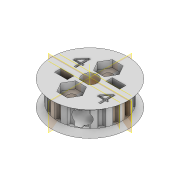
# Autodesk Inventor part: 18 tooth .2 pitch .25 wide belt pulley .25 D bore base
Saved by Autodesk Inventor 2020 (Build 240168000, 168)
## iProperties
Created: 2020-01-17
Part Number: 18 tooth .2 pitch .25 wide belt pulley .25 D bore base
Material: Generic
Document SubType Name: Modeling
Designer: ball
Density: 1 g/cm^3
Appearance: Default
Author: ball
Autodesk Inventor part; units mm, degrees
note: some values were not read from the file. Chosen so that the rebuilt part matches the saved one: direction of "Emboss1".
ref_plane "XZ Plane" through (0, 0, 0) normal (0, 1, 0) x (-1, 0, 0)
sketch "Sketch1" plane through (0, 0, 0) normal (0, 1, 0) x (-1, 0, 0)
  arc A0 (-6.0094, 12.7604) -> (-8.0461, 11.5845) centre (0, 0) ccw
  line L0 (-7.6834, 10.231) -> (-8.0461, 11.5845)
  line L1 (-8.7413, 9.3433) -> (-7.6834, 10.231)
  line L2 (-10.0113, 9.9355) -> (-8.7413, 9.3433)
  arc A1 (-10.0113, 9.9355) -> (-11.523, 8.134) centre (0, 0) ccw
  line L3 (-10.7193, 6.9861) -> (-11.523, 8.134)
  line L4 (-11.4098, 5.7901) -> (-10.7193, 6.9861)
  line L5 (-12.8057, 5.9122) -> (-11.4098, 5.7901)
  arc A2 (-12.8057, 5.9122) -> (-13.6101, 3.7023) centre (0, 0) ccw
  line L6 (-12.4622, 2.8986) -> (-13.6101, 3.7023)
  line L7 (-12.702, 1.5386) -> (-12.4622, 2.8986)
  line L8 (-14.0555, 1.1759) -> (-12.702, 1.5386)
  arc A3 (-14.0555, 1.1759) -> (-14.0555, -1.1759) centre (0, 0) ccw
  line L9 (-12.702, -1.5386) -> (-14.0555, -1.1759)
  line L10 (-12.4622, -2.8986) -> (-12.702, -1.5386)
  line L11 (-13.6101, -3.7023) -> (-12.4622, -2.8986)
  arc A4 (-13.6101, -3.7023) -> (-12.8057, -5.9122) centre (0, 0) ccw
  line L12 (-11.4098, -5.7901) -> (-12.8057, -5.9122)
  line L13 (-10.7193, -6.9861) -> (-11.4098, -5.7901)
  line L14 (-11.523, -8.134) -> (-10.7193, -6.9861)
  arc A5 (-11.523, -8.134) -> (-10.0113, -9.9355) centre (0, 0) ccw
  line L15 (-8.7413, -9.3433) -> (-10.0113, -9.9355)
  line L16 (-7.6834, -10.231) -> (-8.7413, -9.3433)
  line L17 (-8.0461, -11.5845) -> (-7.6834, -10.231)
  arc A6 (-8.0461, -11.5845) -> (-6.0094, -12.7604) centre (0, 0) ccw
  line L18 (-5.0186, -11.7695) -> (-6.0094, -12.7604)
  line L19 (-3.7209, -12.2419) -> (-5.0186, -11.7695)
  line L20 (-3.5987, -13.6378) -> (-3.7209, -12.2419)
  arc A7 (-3.5987, -13.6378) -> (-1.2827, -14.0462) centre (0, 0) ccw
  line L21 (-0.6905, -12.7762) -> (-1.2827, -14.0462)
  line L22 (0.6905, -12.7762) -> (-0.6905, -12.7762)
  line L23 (1.2827, -14.0462) -> (0.6905, -12.7762)
  arc A8 (1.2827, -14.0462) -> (3.5987, -13.6378) centre (0, 0) ccw
  line L24 (3.7209, -12.2419) -> (3.5987, -13.6378)
  line L25 (5.0186, -11.7695) -> (3.7209, -12.2419)
  line L26 (6.0094, -12.7604) -> (5.0186, -11.7695)
  arc A9 (6.0094, -12.7604) -> (8.0461, -11.5845) centre (0, 0) ccw
  line L27 (7.6834, -10.231) -> (8.0461, -11.5845)
  line L28 (8.7413, -9.3433) -> (7.6834, -10.231)
  line L29 (10.0113, -9.9355) -> (8.7413, -9.3433)
  arc A10 (10.0113, -9.9355) -> (11.523, -8.134) centre (0, 0) ccw
  line L30 (10.7193, -6.9861) -> (11.523, -8.134)
  line L31 (11.4098, -5.7901) -> (10.7193, -6.9861)
  line L32 (12.8057, -5.9122) -> (11.4098, -5.7901)
  arc A11 (12.8057, -5.9122) -> (13.6101, -3.7023) centre (0, 0) ccw
  line L33 (12.4622, -2.8986) -> (13.6101, -3.7023)
  line L34 (12.702, -1.5386) -> (12.4622, -2.8986)
  line L35 (14.0555, -1.1759) -> (12.702, -1.5386)
  arc A12 (14.0555, -1.1759) -> (14.0555, 1.1759) centre (0, 0) ccw
  line L36 (12.702, 1.5386) -> (14.0555, 1.1759)
  line L37 (12.4622, 2.8986) -> (12.702, 1.5386)
  line L38 (13.6101, 3.7023) -> (12.4622, 2.8986)
  arc A13 (13.6101, 3.7023) -> (12.8057, 5.9122) centre (0, 0) ccw
  line L39 (11.4098, 5.7901) -> (12.8057, 5.9122)
  line L40 (10.7193, 6.9861) -> (11.4098, 5.7901)
  line L41 (11.523, 8.134) -> (10.7193, 6.9861)
  arc A14 (11.523, 8.134) -> (10.0113, 9.9355) centre (0, 0) ccw
  line L42 (8.7413, 9.3433) -> (10.0113, 9.9355)
  line L43 (7.6834, 10.231) -> (8.7413, 9.3433)
  line L44 (8.0461, 11.5845) -> (7.6834, 10.231)
  arc A15 (8.0461, 11.5845) -> (6.0094, 12.7604) centre (0, 0) ccw
  line L45 (5.0186, 11.7695) -> (6.0094, 12.7604)
  line L46 (3.7209, 12.2419) -> (5.0186, 11.7695)
  line L47 (3.5987, 13.6378) -> (3.7209, 12.2419)
  arc A16 (3.5987, 13.6378) -> (1.2827, 14.0462) centre (0, 0) ccw
  line L48 (0.6905, 12.7762) -> (1.2827, 14.0462)
  line L49 (-0.6905, 12.7762) -> (0.6905, 12.7762)
  line L50 (-1.2827, 14.0462) -> (-0.6905, 12.7762)
  arc A17 (-1.2827, 14.0462) -> (-3.5987, 13.6378) centre (0, 0) ccw
  line L51 (-3.7209, 12.2419) -> (-3.5987, 13.6378)
  line L52 (-5.0186, 11.7695) -> (-3.7209, 12.2419)
  line L53 (-6.0094, 12.7604) -> (-5.0186, 11.7695)
  constraints: 108 end point, 36 point on circle, 18 centre point
extrude "Extrusion1" add sketch "Sketch1" along normal blind 3.4925 and the other way blind 3.4925
sketch "Sketch6" plane through (0, 0, 0) normal (0, 0, 1) x (1, 0, 0)
  line L0 (14.0555, -3.4925) -> (14.1046, -3.4925) projected
  line L1 (14.1046, 3.4925) -> (14.0555, 3.4925) projected
  line L2 (-14.1046, 3.4925) -> (-16.6201, 5.3975)
  line L3 (-14.1046, -3.4925) -> (-16.6201, -5.3975)
  line L4 (11.4098, -3.4925) -> (11.4098, 3.4925) projected
  line L5 (0, 5.3975) -> (-16.6201, 5.3975)
  line L6 (0, -5.3975) -> (-16.6201, -5.3975)
  line L7 (0, -5.3975) -> (0, -3.4925)
  line L8 (-14.1046, -3.4925) -> (0, -3.4925)
  line L9 (0, 5.3975) -> (0, 3.4925)
  line L10 (0, -9.779) -> (0, 9.779) projected
  line L11 (-14.0555, 3.4925) -> (-14.1046, 3.4925) projected
  line L12 (-14.1046, 3.4925) -> (0, 3.4925)
  line L13 (-0.6905, 3.4925) -> (0.6905, 3.4925) projected
  point P0 (0, 0)
  dimension "d34" = 16.6201
  dimension "d36" = 16.6201
  dimension "d73" = 1.905
  dimension "d74" = 1.905
  constraints: 17 end point, 1 collinear, 1 horizontal
  measures "d34" horizontal distance of L2.end point (0, 0)
  measures "d36" horizontal distance of L3.end point (0, 0)
  measures "d73" distance between parallel lines of L8 L6
  measures "d74" distance between parallel lines of L12 L5
revolve "Revolution1" add sketch "Sketch6" angle 360 about axis through (0, 0, 0) along (0, 1, 0)
ref_plane "Work Plane1" through (0, 0, 2.5) normal (0, 0, 1) x (1, 0, 0)
ref_plane "Work Plane2" through (0, 0, -2.5) normal (0, 0, 1) x (1, 0, 0)
sketch "Sketch2" plane through (0, 0, 0) normal (0, 0, 1) x (1, 0, 0)
  circle A0 centre (7.4168, 0) radius 1.7
  circle A1 centre (-7.4168, 0) radius 1.7
  point P0 (0, 0)
  dimension "d5" = 3.4
  dimension "d6" = 7.4168
  dimension "d7" = 3.4
  dimension "d8" = 7.4168
  constraints: 2 centre point
  measures "d5" diameter of A0
  measures "d6" distance of A0.centre point (0, 0)
  measures "d7" diameter of A1
  measures "d8" distance of A1.centre point (0, 0)
extrude "Screw hole 2" cut sketch "Sketch2" along normal blind 2.5 and the other way blind 6 contours A0
sketch "Sketch3" plane through (0, 0, 2.5) normal (0, 0, 1) x (1, 0, 0)
  circle A0 centre (7.4168, 0) radius 1.7 projected
  circle A1 centre (7.4168, 0) radius 3.25
  point P0 (0, 0)
  dimension "d19" = 6.5
  constraints: 1 centre point, 1 coincident
  measures "d19" diameter of A1
sketch "Sketch4" plane through (0, 0, -2.5) normal (0, 0, 1) x (1, 0, 0)
  circle A0 centre (7.4168, 0) radius 1.7 projected
  circle A1 centre (7.4168, 0) radius 3.45 construction
  line L0 (7.4168, -3.45) -> (4.429, -1.725)
  line L1 (4.429, -1.725) -> (4.429, 6.985)
  line L2 (10.4046, 6.985) -> (10.4046, -1.725)
  line L3 (10.4046, -1.725) -> (7.4168, -3.45)
  line L4 (10.4046, 6.985) -> (4.429, 6.985)
  point P0 (0, 0)
  dimension "d22" = 6.9
  constraints: 10 end point, 2 coincident, 1 vertical alignment, 8 other
sketch "Sketch5" plane through (0, 0, -2.5) normal (0, 0, 1) x (1, 0, 0)
  circle A0 centre (-7.422, 0) radius 3.25
  point P0 (0, 0)
  dimension "d25" = 6.5
  constraints: 1 centre point
  measures "d25" diameter of A0
extrude "Access Hole 1" cut sketch "Sketch5" against normal through all
extrude "Access Hole 2" cut sketch "Sketch3" along normal through all contours A0 | A1
extrude "Nut well 2" cut sketch "Sketch4" against normal blind 2.794 contours A0 | L0 L1 L4 L2 L3
sketch "Sketch7" plane through (0, 0, 2.5) normal (0, 0, 1) x (1, 0, 0)
  circle A0 centre (-7.422, 0) radius 3.25 construction
  circle A1 centre (-7.422, 0) radius 3.45 construction
  line L0 (-7.422, -3.25) -> (-10.2365, -1.625)
  line L1 (-10.2365, -1.625) -> (-10.2365, 5.3975)
  line L2 (-4.6074, 5.3975) -> (-4.6074, -1.625)
  line L3 (-4.6074, -1.625) -> (-7.422, -3.25)
  line L4 (16.6201, 5.3975) -> (-16.6201, 5.3975) projected
  line L5 (-10.2365, 5.3975) -> (-4.6074, 5.3975)
  point P0 (0, 0)
  dimension "d48" = 6.9
  constraints: 10 end point, 2 coincident, 2 point on line, 1 centre point, 1 vertical alignment, 7 other
  measures "d48" diameter of A1
extrude "Nut Well 1" cut sketch "Sketch7" along normal blind 2.794
sketch "Sketch8" plane through (0, 0, 0) normal (0, 0, 1) x (1, 0, 0)
  circle A0 centre (-7.422, 0) radius 3.25 projected
  circle A1 centre (-7.422, 0) radius 1.7
  point P0 (0, 0)
  dimension "d51" = 3.4
  constraints: 1 centre point, 1 coincident
  measures "d51" diameter of A1
extrude "Screw Hole 1" cut sketch "Sketch8" along normal blind 6 and the other way blind 2.5 contours A1
sketch "Sketch9" plane through (0, 5.3975, 0) normal (0, 1, 0) x (1, 0, 0)
  arc A0 (1.9431, -2.5908) -> (-1.9431, -2.5908) centre (0, 0) ccw
  line L0 (-1.9431, -2.5908) -> (1.9431, -2.5908)
  dimension "d56" = 6.477
  dimension "d57" = 2.5908
  constraints: 2 end point, 2 point on circle, 1 centre point, 1 coincident, 1 horizontal
  measures "d56" diameter of A0
  measures "d57" distance from line of L0 point (0, 0)
extrude "Center shaft" cut sketch "Sketch9" against normal through all
sketch "Sketch10" plane through (0, 5.3975, 0) normal (0, 1, 0) x (1, 0, 0)
  circle A0 centre (0, 8.001) radius 1.9304
  circle A1 centre (0, -8.001) radius 1.9304
  point P0 (0, 0)
  dimension "d60" = 3.8608
  dimension "d61" = 8.001
  dimension "d62" = 3.8608
  dimension "d63" = 8.001
  constraints: 2 centre point
  measures "d60" diameter of A0
  measures "d61" distance of A0.centre point (0, 0)
  measures "d62" diameter of A1
  measures "d63" distance of A1.centre point (0, 0)
extrude "Wheel holes" cut sketch "Sketch10" against normal through all
sketch "Sketch11" plane through (0, 5.3975, 0) normal (0, 1, 0) x (1, 0, 0)
  circle A0 centre (0, 8.001) radius 1.9304 construction
  circle A1 centre (0, 8.001) radius 4.6609 construction
  circle A2 centre (0, -8.001) radius 1.9304 construction
  circle A3 centre (0, -8.001) radius 4.6482 construction
  line L0 (4.7625, 8.001) -> (2.3813, 3.8766)
  line L1 (2.3813, 3.8766) -> (-2.3812, 3.8766)
  line L2 (-2.3812, 3.8766) -> (-4.7625, 8.001)
  line L3 (-4.7625, 8.001) -> (-2.3813, 12.1254)
  line L4 (-2.3813, 12.1254) -> (2.3812, 12.1254)
  line L5 (2.3812, 12.1254) -> (4.7625, 8.001)
  line L6 (4.7625, -8.001) -> (2.3813, -12.1254)
  line L7 (2.3813, -12.1254) -> (-2.3812, -12.1254)
  line L8 (-2.3812, -12.1254) -> (-4.7625, -8.001)
  line L9 (-4.7625, -8.001) -> (-2.3813, -3.8766)
  line L10 (-2.3813, -3.8766) -> (2.3812, -3.8766)
  line L11 (2.3812, -3.8766) -> (4.7625, -8.001)
  point P0 (0, 0)
  dimension "d67" = 9.3218
  dimension "d68" = 9.2964
  constraints: 24 end point, 4 coincident, 2 centre point, 26 other
  measures "d67" diameter of A1
  measures "d68" diameter of A3
extrude "Wheel hole nut wells" cut sketch "Sketch11" against normal blind 3.048
sketch "Sketch12" plane through (0, 5.3975, 0) normal (0, 1, 0) x (1, 0, 0)
  line L0 (8.4497, -1.4725) -> (12.2618, -1.4725) construction
  line L1 (12.2618, -1.4725) -> (12.2618, -6.5525) construction
  line L2 (12.2618, -6.5525) -> (8.4497, -6.5525) construction
  line L3 (8.4497, -6.5525) -> (8.4497, -1.4725) construction
  line L4 (-11.4769, 8.261) -> (-5.9302, 8.261) construction
  line L5 (-5.9302, 8.261) -> (-5.9302, 0.4721) construction
  line L6 (-5.9302, 0.4721) -> (-11.4769, 0.4721) construction
  line L7 (-11.4769, 0.4721) -> (-11.4769, 8.261) construction
  line L8 (-6.5371, 3.3734) -> (-7.2936, 3.3734)
  line L9 (-7.2936, 3.3734) -> (-7.2936, 1.1915)
  line L10 (-7.2936, 1.1915) -> (-8.1118, 1.1915)
  line L11 (-8.1118, 1.1915) -> (-8.1118, 3.3734)
  line L12 (-8.1118, 3.3734) -> (-10.9163, 3.3734)
  line L13 (-10.9163, 3.3734) -> (-10.9163, 4.2687)
  line L14 (-10.9163, 4.2687) -> (-8.0757, 7.5415)
  line L15 (-8.0757, 7.5415) -> (-7.2936, 7.5415)
  line L16 (-7.2936, 7.5415) -> (-7.2936, 4.0578)
  line L17 (-7.2936, 4.0578) -> (-6.5371, 4.0578)
  line L18 (-6.5371, 4.0578) -> (-6.5371, 3.3734)
  line L19 (-8.1118, 4.0578) -> (-8.1118, 6.5381)
  line L20 (-8.1118, 6.5381) -> (-10.2473, 4.0578)
  line L21 (-10.2473, 4.0578) -> (-8.1118, 4.0578)
  line L22 (12.5221, -5.0056) -> (11.7657, -5.0056)
  line L23 (11.7657, -5.0056) -> (11.7657, -7.1875)
  line L24 (11.7657, -7.1875) -> (10.9475, -7.1875)
  line L25 (10.9475, -7.1875) -> (10.9475, -5.0056)
  line L26 (10.9475, -5.0056) -> (8.143, -5.0056)
  line L27 (8.143, -5.0056) -> (8.143, -4.1102)
  line L28 (8.143, -4.1102) -> (10.9835, -0.8375)
  line L29 (10.9835, -0.8375) -> (11.7657, -0.8375)
  line L30 (11.7657, -0.8375) -> (11.7657, -4.3212)
  line L31 (11.7657, -4.3212) -> (12.5221, -4.3212)
  line L32 (12.5221, -4.3212) -> (12.5221, -5.0056)
  line L33 (10.9475, -4.3212) -> (10.9475, -1.8409)
  line L34 (10.9475, -1.8409) -> (8.812, -4.3212)
  line L35 (8.812, -4.3212) -> (10.9475, -4.3212)
  point P0 (0, 0)
  constraints: 4 other
emboss "Emboss1" sketch "Sketch12" operation cut depth 0.635 direction (0, -1, 0)
equation "\"d34\" = d32"
equation "\"d36\" = d32"
equation "\"d74\" = d73"
equation "\"d32\" = 16.620096"
body "Solid1"
